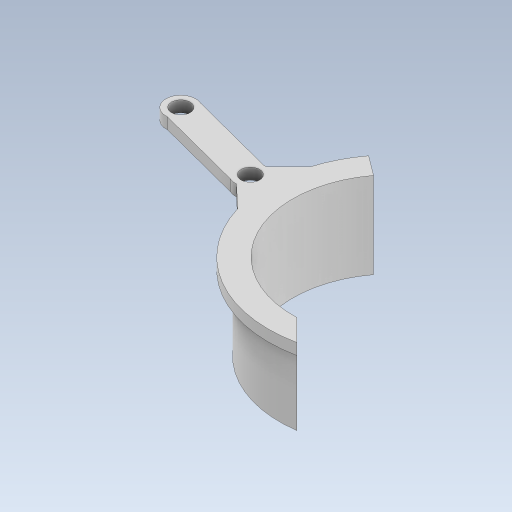
# Autodesk Inventor part: Left Hand
Saved by Autodesk Inventor 2023.5 (Build 275446000, 446)
## iProperties
Created: 2025-10-05
Part Number: Left Hand
Material: Generic
Document SubType Name: Modeling
Designer: Guntur
Density: 1 g/cm^3
Appearance: Default
Author: Guntur
## iProperties of the stored document Left Hand_3DPrint.ipt
Created: 2025-10-05
Part Number: Left Hand_3DPrint
Material: Generic
Document SubType Name: Modeling
Designer: Guntur
Density: 1 g/cm^3
Appearance: Default
Author: Guntur
Autodesk Inventor part; units mm, degrees
ref_plane "YZ Plane" through (0, 0, 0) normal (1, 0, 0) x (0, 1, 0)
ref_plane "XZ Plane" through (0, 0, 0) normal (0, 1, 0) x (-1, 0, 0)
ref_plane "XY Plane" through (0, 0, 0) normal (0, 0, 1) x (1, 0, 0)
sketch "Sketch1" plane through (0, 0, 0) normal (0, 1, 0) x (-1, 0, 0)
  circle A0 centre (38.808, -218.8887) radius 2.5
  circle A1 centre (38.808, -218.8887) radius 4
  line L0 (38.5178, -214.8993) -> (32.6339, -209.3346)
  line L1 (38.5178, -222.8782) -> (32.6339, -228.6797)
  line L2 (38.5178, -214.8993) -> (44.821, -214.8993) construction
  line L3 (36.4862, -222.1459) -> (62.0591, -228.8274)
  line L4 (63.7262, -225.1914) -> (63.7262, -218.8414)
  line L5 (38.808, -218.8887) -> (63.7262, -225.1914)
  circle A2 centre (63.7262, -225.1914) radius 2.5
  circle A3 centre (63.7262, -225.1914) radius 4
  line L6 (66.048, -221.9342) -> (40.4751, -215.2527)
  line L7 (38.5178, -222.8782) -> (46.8388, -222.8782) construction
  arc A4 (23.7643, -236.4024) -> (-22.704, -201.6938) centre (0.5607, -219.0071) ccw
  arc A5 (24.9661, -237.3) -> (-23.9058, -200.7962) centre (0.5607, -219.0071) ccw
  arc A6 (27.3696, -239.0953) -> (-26.3093, -199.0009) centre (0.5607, -219.0071) ccw
  line L8 (0.5607, -219.0071) -> (33.0607, -219.0071) construction
  line L9 (-11.1066, -187.6045) -> (-8.0218, -191.3062)
  line L10 (27.3696, -239.0953) -> (-26.3093, -199.0009)
  circle A7 centre (0.5607, -219.0071) radius 27
  line L11 (-8.0218, -191.3062) -> (-6.6103, -193)
  line L12 (-26.3093, -199.0009) -> (-26.3093, -179)
  line L13 (-26.3093, -179) -> (-6.3093, -179)
  line L14 (-6.3093, -179) -> (-6.3093, -186.2191)
  line L15 (-6.3093, -186.2191) -> (-1.2222, -191.3062)
  line L16 (-6.3093, -186.2191) -> (0.8849, -186.2191) construction
  line L17 (-1.2222, -191.3062) -> (-0.5005, -192.028)
  point P0 (35.5254, -216.603)
  point P1 (34.0607, -219.0071)
  point P2 (33.8894, -222.3906)
  point P3 (23.4919, -219.4969)
  point P4 (-23.1273, -195.3191)
  point P5 (24.2488, -242.6952)
  point P6 (39.2399, -222.8653)
  point P7 (63.2943, -221.2147)
  point P8 (-9.0575, -190.0634)
  point P9 (-6.626, -192.9812)
  point P10 (22.1619, -235.2055)
  point P11 (-3.7195, -188.809)
  dimension "d48" = 33.5
  dimension "d59" = 54
  dimension "d47" = 5
  dimension "d49" = 30.5
  dimension "d50" = 29
  dimension "d51" = 66.9999
  dimension "d52" = 5.8838
  dimension "d53" = 5.8838
  dimension "d54" = 25.5729
  dimension "d55" = 25.5729
  dimension "d56" = 8
  dimension "d57" = 5
  dimension "d58" = 8
  dimension "d60" = 20
  dimension "d61" = 45
  constraints: 36 end point, 12 point on circle, 6 centre point, 6 coincident, 5 point on line, 2 perpendicular, 1 equal length, 1 horizontal, 1 vertical, 15 other
  measures "d47" diameter of A0
  measures "d49" radius of A5
  measures "d50" radius of A4
  measures "d51" distance of L10.start L10.end
  measures "d52" horizontal distance of L7.start L1.end
  measures "d53" horizontal distance of L0.start L0.end
  measures "d54" horizontal distance of L3.start L3.end
  measures "d55" horizontal distance of L6.start L6.end
  measures "d56" diameter of A3
  measures "d57" diameter of A2
  measures "d58" diameter of A1
  measures "d60" distance of L12.end L13.end
  measures "d61" angle of L15 L16
extrude "Extrusion5" add sketch "Sketch1" along normal blind 3 contours A1 L3 | A1 L6 A3 L5 | L5 A3 L3 A1 | A1 L3 | A3 L6 L4 A2 L5 | L5 A2 L4 L6 A3 | L1 A6 L0 A1 | A3 L4 L6 | A6 L10 A5 L15 | A3 L6 L4
extrude "Extrusion6" add sketch "Sketch1" along normal blind 3 and the other way blind 20 contours L10 A4 L15 A5 | L10 A7 L17 L15 A4
body "Solid3"
